Autodesk Inventor part; units mm, degrees
(part 2 of 2)
  arc A205 (-7.2812, 208.5616) -> (-8.6448, 208.5044) centre (-6.6997, 178.392) ccw projected
  arc A206 (-8.6448, 208.5044) -> (-9.6498, 211.2799) centre (-21.0077, 205.5976) ccw projected
  arc A207 (-9.6498, 211.2799) -> (-10.6519, 211.1746) centre (-6.6997, 178.392) ccw projected
  arc A208 (-10.6519, 211.1746) -> (-11.0579, 208.2508) centre (1.6392, 207.9779) ccw projected
  arc A209 (-11.0579, 208.2508) -> (-12.4036, 208.0232) centre (-6.6997, 178.392) ccw projected
  arc A210 (-12.4036, 208.0232) -> (-13.7485, 210.6508) centre (-24.3047, 203.5899) ccw projected
  arc A211 (-13.7485, 210.6508) -> (-14.7295, 210.4207) centre (-6.6997, 178.392) ccw projected
  arc A212 (-14.7295, 210.4207) -> (-14.7658, 207.4691) centre (-2.1347, 208.7898) ccw projected
  arc A213 (-14.7658, 207.4691) -> (-16.0724, 207.0746) centre (-6.6997, 178.392) ccw projected
  arc A214 (-16.0724, 207.0746) -> (-17.736, 209.513) centre (-27.324, 201.1847) ccw projected
  arc A215 (-17.736, 209.513) -> (-18.6805, 209.1618) centre (-6.6997, 178.392) ccw projected
  arc A216 (-18.6805, 209.1618) -> (-18.3466, 206.2289) centre (-5.9806, 209.1222) ccw projected
  arc A217 (-18.3466, 206.2289) -> (-19.5934, 205.6738) centre (-6.6997, 178.392) ccw projected
  arc A218 (-19.5934, 205.6738) -> (-21.5495, 207.8844) centre (-30.018, 198.4201) ccw projected
  arc A219 (-21.5495, 207.8844) -> (-22.4425, 207.4176) centre (-6.6997, 178.392) ccw projected
  arc A220 (-22.4425, 207.4176) -> (-21.7436, 204.5496) centre (-9.8377, 208.9701) ccw projected
  arc A221 (-21.7436, 204.5496) -> (-22.911, 203.8426) centre (-6.6997, 178.392) ccw projected
  arc A222 (-22.911, 203.8426) -> (-25.1288, 205.7907) centre (-32.3443, 195.3396) ccw projected
  arc A223 (-25.1288, 205.7907) -> (-25.9562, 205.2156) centre (-6.6997, 178.392) ccw projected
  arc A224 (-25.9562, 205.2156) -> (-24.9034, 202.4579) centre (-13.6455, 208.3356) ccw projected
  arc A225 (-24.9034, 202.4579) -> (-25.973, 201.6101) centre (-6.6997, 178.392) ccw projected
  arc A226 (-25.973, 201.6101) -> (-28.4175, 203.2649) centre (-34.2662, 191.9918) ccw projected
  arc A227 (-28.4175, 203.2649) -> (-29.1663, 202.5906) centre (-6.6997, 178.392) ccw projected
  arc A228 (-29.1663, 202.5906) -> (-27.7761, 199.9866) centre (-17.3436, 207.229) ccw projected
  arc A229 (-27.7761, 199.9866) -> (-28.731, 199.0115) centre (-6.6997, 178.392) ccw projected
  arc A230 (-28.731, 199.0115) -> (-31.3636, 200.3468) centre (-35.7534, 188.4296) ccw projected
  arc A231 (-31.3636, 200.3468) -> (-32.022, 199.584) centre (-6.6997, 178.392) ccw projected
  arc A232 (-32.022, 199.584) -> (-30.3165, 197.1747) centre (-20.8739, 205.6676) ccw projected
  arc A233 (-30.3165, 197.1747) -> (-31.1416, 196.0876) centre (-6.6997, 178.392) ccw projected
  arc A234 (-31.1416, 196.0876) -> (-33.9208, 197.0825) centre (-36.7823, 184.709) ccw projected
  arc A235 (-33.9208, 197.0825) -> (-34.4784, 196.2432) centre (-6.6997, 178.392) ccw projected
  arc A236 (-34.4784, 196.2432) -> (-32.4844, 194.0667) centre (-24.1807, 203.676) ccw projected
  arc A237 (-32.4844, 194.0667) -> (-33.1668, 192.8847) centre (-6.6997, 178.392) ccw projected
  arc A238 (-33.1668, 192.8847) -> (-36.0487, 193.5234) centre (-37.3369, 180.8889) ccw projected
  arc A239 (-36.0487, 193.5234) -> (-36.4967, 192.6208) centre (-6.6997, 178.392) ccw projected
  arc A240 (-36.4967, 192.6208) -> (-34.2456, 190.7114) centre (-27.2118, 201.2857) ccw projected
  arc A241 (-34.2456, 190.7114) -> (-34.7745, 189.4533) centre (-6.6997, 178.392) ccw projected
  arc A242 (-34.7745, 189.4533) -> (-37.7137, 189.7257) centre (-37.4082, 177.0293) ccw projected
  arc A243 (-37.7137, 189.7257) -> (-38.0451, 188.7741) centre (-6.6997, 178.392) ccw projected
  arc A244 (-38.0451, 188.7741) -> (-35.5724, 187.1618) centre (-29.9194, 198.5343) ccw projected
  arc A245 (-35.5724, 187.1618) -> (-35.9394, 185.8473) centre (-6.6997, 178.392) ccw projected
  arc A246 (-35.9394, 185.8473) -> (-38.8897, 185.7492) centre (-36.9953, 173.1913) ccw projected
  arc A247 (-38.8897, 185.7492) -> (-39.0992, 184.7636) centre (-6.6997, 178.392) ccw projected
  arc A248 (-39.0992, 184.7636) -> (-36.4439, 183.474) centre (-32.2608, 195.4653) ccw projected
  arc A249 (-36.4439, 183.474) -> (-36.6433, 182.1238) centre (-6.6997, 178.392) ccw projected
  arc A250 (-36.6433, 182.1238) -> (-39.558, 181.6567) centre (-36.1046, 169.4353) ccw projected
  arc A251 (-39.558, 181.6567) -> (-39.6423, 180.6526) centre (-6.6997, 178.392) ccw projected
  arc A252 (-39.6423, 180.6526) -> (-36.8463, 179.706) centre (-34.1991, 192.127) ccw projected
  arc A253 (-36.8463, 179.706) -> (-36.8749, 178.3415) centre (-6.6997, 178.392) ccw projected
  arc A254 (-36.8749, 178.3415) -> (-39.708, 177.5128) centre (-34.7502, 165.8205) ccw projected
  arc A255 (-39.708, 177.5128) -> (-39.6658, 176.506) centre (-6.6997, 178.392) ccw projected
  arc A256 (-39.6658, 176.506) -> (-36.7733, 175.9172) centre (-35.7037, 188.5721) ccw projected
  arc A257 (-36.7733, 175.9172) -> (-36.6306, 174.5599) centre (-6.6997, 178.392) ccw projected
  arc A258 (-36.6306, 174.5599) -> (-39.3376, 173.3827) centre (-32.9533, 162.404) ccw projected
  arc A259 (-39.3376, 173.3827) -> (-39.1695, 172.3891) centre (-6.6997, 178.392) ccw projected
  arc A260 (-39.1695, 172.3891) -> (-36.226, 172.1675) centre (-36.7509, 184.8567) ccw projected
  arc A261 (-36.226, 172.1675) -> (-35.9143, 170.8388) centre (-6.6997, 178.392) ccw projected
  arc A262 (-35.9143, 170.8388) -> (-38.4524, 169.3316) centre (-30.7425, 159.2396) ccw projected
  arc A263 (-38.4524, 169.3316) -> (-38.1611, 168.3669) centre (-6.6997, 178.392) ccw projected
  arc A264 (-38.1611, 168.3669) -> (-35.2131, 168.516) centre (-37.3242, 181.0393) ccw projected
  arc A265 (-35.2131, 168.516) -> (-34.7373, 167.2368) centre (-6.6997, 178.392) ccw projected
  arc A266 (-34.7373, 167.2368) -> (-37.0664, 165.4233) centre (-28.1525, 156.3773) ccw projected
  arc A267 (-37.0664, 165.4233) -> (-36.6566, 164.5028) centre (-6.6997, 178.392) ccw projected
  arc A268 (-36.6566, 164.5028) -> (-33.7504, 165.0202) centre (-37.4145, 177.1802) ccw projected
  arc A269 (-33.7504, 165.0202) -> (-33.1181, 163.8107) centre (-6.6997, 178.392) ccw projected
  arc A270 (-33.1181, 163.8107) -> (-35.2016, 161.7197) centre (-25.2242, 153.8621) ccw projected
  arc A271 (-35.2016, 161.7197) -> (-34.6796, 160.8577) centre (-6.6997, 178.392) ccw projected
  arc A272 (-34.6796, 160.8577) -> (-31.8612, 161.7353) centre (-37.0205, 173.3401) ccw projected
  arc A273 (-31.8612, 161.7353) -> (-31.0823, 160.6146) centre (-6.6997, 178.392) ccw projected
  arc A274 (-31.0823, 160.6146) -> (-32.8872, 158.2789) centre (-22.0037, 151.7338) ccw projected
  arc A275 (-32.8872, 158.2789) -> (-32.2613, 157.4892) centre (-6.6997, 178.392) ccw projected
  arc A276 (-32.2613, 157.4892) -> (-29.5752, 158.7131) centre (-36.1482, 169.5798) ccw projected
  arc A277 (-29.5752, 158.7131) -> (-28.6619, 157.6989) centre (-6.6997, 178.392) ccw projected
  arc A278 (-28.6619, 157.6989) -> (-30.1599, 155.1553) centre (-18.5419, 150.0259) ccw projected
  arc A279 (-30.1599, 155.1553) -> (-29.44, 154.4503) centre (-6.6997, 178.392) ccw projected
  arc A280 (-29.44, 154.4503) -> (-26.9284, 156.0012) centre (-34.8116, 165.9584) ccw projected
  arc A281 (-26.9284, 156.0012) -> (-25.8952, 155.1094) centre (-6.6997, 178.392) ccw projected
  arc A282 (-25.8952, 155.1094) -> (-27.0626, 152.3982) centre (-14.8933, 148.7654) ccw projected
  arc A283 (-27.0626, 152.3982) -> (-26.26, 151.789) centre (-6.6997, 178.392) ccw projected
  arc A284 (-26.26, 151.789) -> (-23.9626, 153.6424) centre (-33.0315, 162.5331) ccw projected
  arc A285 (-23.9626, 153.6424) -> (-22.8258, 152.8872) centre (-6.6997, 178.392) ccw projected
  arc A286 (-22.8258, 152.8872) -> (-23.6442, 150.051) centre (-11.1155, 147.9721) ccw projected
  arc A287 (-23.6442, 150.051) -> (-22.7715, 149.5472) centre (-6.6997, 178.392) ccw projected
  arc A288 (-22.7715, 149.5472) -> (-20.7245, 151.674) centre (-30.8363, 159.3579) ccw projected
  arc A289 (-20.7245, 151.674) -> (-19.502, 151.0672) centre (-6.6997, 178.392) ccw projected
  arc A290 (-19.502, 151.0672) -> (-19.9585, 148.1508) centre (-7.268, 147.6585) ccw projected
  arc A291 (-19.9585, 148.1508) -> (-19.0296, 147.7603) centre (-6.6997, 178.392) ccw projected
  arc A292 (-19.0296, 147.7603) -> (-17.2653, 150.1269) centre (-28.2603, 156.4829) ccw projected
  arc A293 (-17.2653, 150.1269) -> (-15.9764, 149.6781) centre (-6.6997, 178.392) ccw projected
  arc A294 (-15.9764, 149.6781) -> (-16.0637, 146.7275) centre (-3.4116, 147.8296) ccw projected
  arc A295 (-16.0637, 146.7275) -> (-15.0932, 146.4565) centre (-6.6997, 178.392) ccw projected
  arc A296 (-15.0932, 146.4565) -> (-13.6394, 149.0256) centre (-25.3444, 153.9534) ccw projected
  arc A297 (-13.6394, 149.0256) -> (-12.3044, 148.7418) centre (-6.6997, 178.392) ccw projected
  arc A298 (-12.3044, 148.7418) -> (-12.0213, 145.8036) centre (0.3929, 148.4827) ccw projected
  arc A299 (-12.0213, 145.8036) -> (-11.0244, 145.6564) centre (-6.6997, 178.392) ccw projected
  arc A300 (-11.0244, 145.6564) -> (-9.9041, 148.3874) centre (-22.1344, 151.8093) ccw projected
  arc A301 (-9.9041, 148.3874) -> (-8.5441, 148.2732) centre (-6.6997, 178.392) ccw projected
  arc A302 (-8.5441, 148.2732) -> (-7.8949, 145.3936) centre (4.0856, 149.6075) ccw projected
  arc A303 (-7.8949, 145.3936) -> (-6.8875, 145.3725) centre (-6.6997, 178.392) ccw projected
  arc A304 (-6.8875, 145.3725) -> (-6.1183, 148.2224) centre (-18.681, 150.0844) ccw projected
  arc A305 (-6.1183, 148.2224) -> (-4.7547, 148.2795) centre (-6.6997, 178.392) ccw projected
  arc A306 (-4.7547, 148.2795) -> (-3.7497, 145.504) centre (7.6082, 151.1863) ccw projected
  arc A307 (-3.7497, 145.504) -> (-2.7476, 145.6093) centre (-6.6997, 178.392) ccw projected
  arc A308 (-2.7476, 145.6093) -> (-2.3416, 148.5331) centre (-15.0387, 148.806) ccw projected
  arc A309 (-2.3416, 148.5331) -> (-0.9959, 148.7607) centre (-6.6997, 178.392) ccw projected
  arc A310 (-0.9959, 148.7607) -> (0.349, 146.1331) centre (10.9052, 153.1941) ccw projected
  arc A311 (0.349, 146.1331) -> (1.33, 146.3632) centre (-6.6997, 178.392) ccw projected
  arc A312 (1.33, 146.3632) -> (1.3663, 149.3148) centre (-11.2648, 147.9941) ccw projected
  arc A313 (1.3663, 149.3148) -> (2.6729, 149.7093) centre (-6.6997, 178.392) ccw projected
  arc A314 (2.6729, 149.7093) -> (4.3365, 147.2709) centre (13.9245, 155.5992) ccw projected
  arc A315 (4.3365, 147.2709) -> (5.281, 147.6221) centre (-6.6997, 178.392) ccw projected
  arc A316 (5.281, 147.6221) -> (4.9471, 150.555) centre (-7.4189, 147.6617) ccw projected
  arc A317 (4.9471, 150.555) -> (6.1939, 151.1101) centre (-6.6997, 178.392) ccw projected
  arc A318 (6.1939, 151.1101) -> (8.15, 148.8995) centre (16.6185, 158.3639) ccw projected
  arc A319 (8.15, 148.8995) -> (9.043, 149.3663) centre (-6.6997, 178.392) ccw projected
  arc A320 (9.043, 149.3663) -> (8.3441, 152.2343) centre (-3.5618, 147.8139) ccw projected
  arc A321 (8.3441, 152.2343) -> (9.5115, 152.9413) centre (-6.6997, 178.392) ccw projected
  arc A322 (9.5115, 152.9413) -> (11.7293, 150.9932) centre (18.9448, 161.4443) ccw projected
  arc A323 (11.7293, 150.9932) -> (12.5567, 151.5683) centre (-6.6997, 178.392) ccw projected
  arc A324 (12.5567, 151.5683) -> (11.5039, 154.326) centre (0.246, 148.4483) ccw projected
  arc A325 (11.5039, 154.326) -> (12.5735, 155.1738) centre (-6.6997, 178.392) ccw projected
  arc A326 (12.5735, 155.1738) -> (15.018, 153.519) centre (20.8667, 164.7921) ccw projected
  arc A327 (15.018, 153.519) -> (15.7668, 154.1933) centre (-6.6997, 178.392) ccw projected
  arc A328 (15.7668, 154.1933) -> (14.3766, 156.7973) centre (3.9441, 149.5549) ccw projected
  arc A329 (14.3766, 156.7973) -> (15.3315, 157.7724) centre (-6.6997, 178.392) ccw projected
  arc A330 (15.3315, 157.7724) -> (17.9641, 156.4371) centre (22.3539, 168.3543) ccw projected
  arc A331 (17.9641, 156.4371) -> (18.6225, 157.1999) centre (-6.6997, 178.392) ccw projected
  arc A332 (18.6225, 157.1999) -> (16.917, 159.6092) centre (7.4744, 151.1163) ccw projected
  arc A333 (16.917, 159.6092) -> (17.7421, 160.6963) centre (-6.6997, 178.392) ccw projected
  arc A334 (17.7421, 160.6963) -> (20.5213, 159.7014) centre (23.3828, 172.0749) ccw projected
  arc A335 (20.5213, 159.7014) -> (21.0789, 160.5407) centre (-6.6997, 178.392) ccw projected
  arc A336 (21.0789, 160.5407) -> (19.0849, 162.7172) centre (10.7812, 153.1079) ccw projected
  arc A337 (19.0849, 162.7172) -> (19.7673, 163.8992) centre (-6.6997, 178.392) ccw projected
  arc A338 (19.7673, 163.8992) -> (22.6492, 163.2605) centre (23.9374, 175.895) ccw projected
  arc A339 (22.6492, 163.2605) -> (23.0972, 164.1631) centre (-6.6997, 178.392) ccw projected
  arc A340 (23.0972, 164.1631) -> (20.8461, 166.0725) centre (13.8123, 155.4982) ccw projected
  arc A341 (20.8461, 166.0725) -> (21.375, 167.3307) centre (-6.6997, 178.392) ccw projected
  line L3 (61.9125, 171.704) -> (29.446, 168.6111) projected
  circle A342 centre (-6.6997, 178.392) radius 37.4457
  circle A343 centre (36.5125, 146.05) radius 28.194
  point P0 (0, 0)
  point P1 (50.3685, 170.6043)
  point P2 (30.4357, 173.5813)
  dimension "d10" = 56.388
  constraints: 2 coincident, 1 centre point, 3 other
  measures "d10" diameter of A343
extrude "Extrusion2" cut sketch "Sketch2" against normal blind 12.7 contours A343 L3 A342
sketch "Sketch3" plane through (0, 0, 0) normal (0, 0, -1) x (-1, 0, 0)
  arc A0 (50.3685, 170.6043) -> (30.4357, 173.5813) centre (36.5125, 146.05) ccw projected
  line L0 (61.9125, 171.704) -> (50.3685, 170.6043) projected
  line L1 (61.9125, 190.5) -> (61.9125, 171.704) projected
  arc A1 (40.9534, 289.0612) -> (-0.498, 261.4395) centre (17.4625, 279.4) ccw projected
  circle A2 centre (17.4625, 279.4) radius 15.9004 projected
  circle A3 centre (40.0964, 179.0237) radius 3.175 projected
  circle A4 centre (52.7964, 180.2336) radius 3.175 projected
  circle A5 centre (40.0964, 182.1987) radius 3.175
  arc A6 (29.446, 168.6111) -> (30.4357, 173.5813) centre (-6.6997, 178.392) ccw projected
  point P0 (0, 0)
  point P1 (42.8461, 180.6112)
  point P2 (37.3468, 180.6112)
  dimension "d13" = 6.35
  constraints: 1 centre point, 4 other
  measures "d13" diameter of A5
extrude "Extrusion3" add sketch "Sketch3" against normal blind 12.7 contours A3 A5 picked at (39.9369, 176.9303)
extrude "Extrusion4" cut sketch "Sketch3" against normal blind 12.7 contours A3 A5 picked at (39.9369, 184.2921)
fillet "Fillet1" radius 6.35 2 edges at (-50.3685, 170.6043, 6.35) (-61.9125, 171.704, 6.35)
sketch "Sketch4" plane through (0, 0, 0) normal (0, 0, -1) x (-1, 0, 0)
  arc A0 (56.1647, 171.1564) -> (61.9125, 177.4778) centre (55.5625, 177.4778) ccw projected
  line L0 (61.9125, 190.5) -> (61.9125, 177.4778) projected
  spline S0 degree 2 poles (40.9534, 289.0612) (61.9125, 238.0996) (61.9125, 190.5) knots 0 0 0 1 1 1
  arc A1 (40.9534, 289.0612) -> (-0.498, 261.4395) centre (17.4625, 279.4) ccw projected
  spline S1 degree 3 poles (29.446, 168.6111) (27.6192, 182.9318) (26.9203, 234.0212) (-0.498, 261.4395) knots 0 0 0 0 1 1 1 1
  arc A2 (48.8612, 171.3959) -> (30.4357, 173.5813) centre (36.5125, 146.05) ccw projected
  arc A3 (48.8612, 171.3959) -> (52.2446, 170.783) centre (51.6424, 177.1044) ccw projected
  line L1 (56.1647, 171.1564) -> (52.2446, 170.783) projected
  circle A4 centre (17.4625, 279.4) radius 15.9004 projected
  circle A5 centre (40.0964, 182.1987) radius 3.175 projected
  circle A6 centre (52.7964, 180.2336) radius 3.175 projected
  line L2 (55.5625, 190.5) -> (55.5625, 177.4778)
  line L3 (55.5625, 177.4778) -> (51.6424, 177.1044)
  arc A7 (51.6424, 177.1044) -> (34.6938, 180.5461) centre (36.5125, 146.05) ccw
  arc A8 (35.0807, 286.6459) -> (3.9921, 265.9296) centre (17.4625, 279.4) ccw
  circle A9 centre (17.4625, 279.4) radius 40.9661
  circle A10 centre (40.0964, 182.1987) radius 9.525
  circle A11 centre (52.7964, 180.2336) radius 9.525
  line L4 (33.448, 192.2945) -> (55.5625, 190.5)
  line L5 (47.1822, 251.2049) -> (33.448, 192.2945)
  line L6 (50.6373, 249.2445) -> (38.1622, 195.7345)
  line L7 (38.1622, 195.7345) -> (59.3725, 194.0133)
  line L8 (59.3725, 194.0133) -> (59.3725, 174.0135)
  line L9 (59.3725, 174.0135) -> (50.9032, 173.2067)
  arc A12 (50.9032, 173.2067) -> (37.3679, 176.7721) centre (36.5125, 146.05) ccw
  line L10 (44.4515, 250.6867) -> (30.3031, 189.9997)
  line L11 (30.3031, 189.9997) -> (53.0208, 188.1562)
  line L12 (53.0208, 188.1562) -> (53.0208, 179.7889)
  line L13 (53.0208, 179.7889) -> (52.0994, 179.7012)
  arc A13 (52.0994, 179.7012) -> (37.5447, 183.1214) centre (36.5125, 146.05) ccw
  arc A14 (29.446, 168.6111) -> (30.4357, 173.5813) centre (-6.6997, 178.392) ccw projected
  spline S2 degree 5 poles (34.6938, 180.5461) (34.5354, 182.2782) (34.3709, 184.0098) (34.1972, 185.7405) (33.7041, 190.3635) (33.1253, 194.9769) (32.7234, 197.8591) (31.7796, 203.9538) (30.6206, 210.0115) (29.9427, 213.1978) (28.398, 219.7282) (26.5193, 226.1708) (25.4561, 229.457) (23.0874, 236.0456) (20.2467, 242.4451) (18.6762, 245.628) (15.2193, 251.9029) (11.1499, 257.7995) (8.9323, 260.6586) (6.5449, 263.3768) (3.9921, 265.9296) knots 0 0 0 0 0 0 0.093954 0.093954 0.093954 0.25113 0.25113 0.25113 0.427044 0.427044 0.427044 0.6135 0.6135 0.6135 0.804991 0.804991 0.804991 1 1 1 1 1 1
  spline S3 degree 5 poles (35.0807, 286.6459) (42.6076, 268.3457) (48.7539, 249.483) (53.2276, 230.0774) (55.5632, 210.2861) (55.5625, 190.5) knots 0 0 0 0 0 0 1 1 1 1 1 1
  point P0 (0, 0)
  point P1 (32.4777, 199.3272)
  point P2 (43.8377, 248.054)
  point P3 (21.8585, 238.6704)
  point P4 (55.5277, 194.3253)
  point P5 (49.2184, 243.1584)
  dimension "d19" = 6.35
  dimension "d20" = 19.05
  dimension "d21" = 19.05
  dimension "d22" = 3.81
  constraints: 24 end point, 8 point on circle, 6 centre point, 3 coincident, 3 concentric, 1 tangent, 23 other
  measures "d20" diameter of A10
  measures "d21" diameter of A11
  measures "d22" distance between parallel lines of L5 L6
extrude "Extrusion5" cut sketch "Sketch4" against normal blind 12.7 contours L7 L6 S3 | L10 S2 A9
fillet "Fillet2" radius 3.175 6 edges at (-43.8377, 248.054, 6.35) (-49.2184, 243.1584, 6.35) (-21.8585, 238.6704, 6.35) (-32.4777, 199.3272, 6.35) (-38.1622, 195.7345, 6.35) (-55.5278, 194.3253, 6.35)
thread "Thread1" size "1/4-20 UNC" class "2B" standard "ANSI Unified Screw Threads" full length
thread "Thread2" size "8-32 UNC" class "2B" standard "ANSI Unified Screw Threads" full length
sketch "Sketch5" plane through (0, 0, 0) normal (0, 0, -1) x (-1, 0, 0)
  circle A0 centre (52.7964, 180.2336) radius 3.175 projected
  circle A1 centre (52.7964, 180.2336) radius 2.413
  circle A2 centre (40.0964, 182.1987) radius 3.175 projected
  circle A3 centre (40.0964, 182.1987) radius 2.413
  point P0 (0, 0)
  dimension "d30" = 4.826
  dimension "d31" = 4.826
  constraints: 2 centre point, 2 coincident
  measures "d30" diameter of A1
  measures "d31" diameter of A3
extrude "Extrusion6" add sketch "Sketch5" against normal blind 12.7
thread "Thread3" size "10-24 UNC" class "2B" standard "ANSI Unified Screw Threads" full length
thread "Thread4" size "10-24 UNC" class "2B" standard "ANSI Unified Screw Threads" full length
sketch "Sketch6" plane through (0, 0, 12.7) normal (0, 0, 1) x (1, 0, 0)
  circle A0 centre (-40.0964, 182.1987) radius 2.413 projected
  circle A1 centre (-52.7964, 180.2336) radius 2.413 projected
  line L0 (-35.8997, 214.0052) -> (-41.9802, 240.0866) projected
  arc A2 (-37.347, 243.5834) -> (-41.9802, 240.0866) centre (-38.8881, 240.8075) ccw projected
  arc A3 (-37.347, 243.5834) -> (-25.6845, 239.2675) centre (-17.4625, 279.4) ccw projected
  line L1 (-45.9336, 229.0686) -> (-38.9986, 199.3221) projected
  arc A4 (-41.8339, 195.4366) -> (-38.9986, 199.3221) centre (-42.0907, 198.6012) ccw projected
  line L2 (-41.8339, 195.4366) -> (-52.0034, 194.6113) projected
  arc A5 (-61.9125, 177.4778) -> (-56.1647, 171.1564) centre (-55.5625, 177.4778) ccw projected
  line L3 (-56.1647, 171.1564) -> (-52.2446, 170.783) projected
  arc A6 (-52.2446, 170.783) -> (-48.8612, 171.3959) centre (-51.6424, 177.1044) ccw projected
  arc A7 (-30.4357, 173.5813) -> (-48.8612, 171.3959) centre (-36.5125, 146.05) ccw projected
  arc A8 (0.498, 261.4395) -> (-40.9534, 289.0612) centre (-17.4625, 279.4) ccw projected
  line L4 (-61.9125, 190.5) -> (-61.9125, 177.4778) projected
  circle A9 centre (-17.4625, 279.4) radius 15.9004 projected
  circle A10 centre (-52.7964, 180.2336) radius 1.27
  circle A11 centre (-40.0964, 182.1987) radius 1.27
  arc A12 (-30.4357, 173.5813) -> (-29.446, 168.6111) centre (6.6997, 178.392) ccw projected
  point P0 (0, 0)
  dimension "d38" = 2.54
  dimension "d39" = 2.54
  constraints: 2 centre point, 2 coincident, 8 other
  measures "d38" diameter of A10
  measures "d39" diameter of A11
extrude "Extrusion7" add sketch "Sketch6" against normal up to surface (12.7 mm away) contours A0 | A1
sketch "Sketch7" plane through (0, 0, 12.7) normal (0, 0, 1) x (1, 0, 0)
  circle A0 centre (-40.0964, 182.1987) radius 1.27 projected
  circle A1 centre (-52.7964, 180.2336) radius 1.27 projected
  line L0 (-35.8997, 214.0052) -> (-41.9802, 240.0866) projected
  arc A2 (-37.347, 243.5834) -> (-41.9802, 240.0866) centre (-38.8881, 240.8075) ccw projected
  arc A3 (-37.347, 243.5834) -> (-25.6845, 239.2675) centre (-17.4625, 279.4) ccw projected
  line L1 (-45.9336, 229.0686) -> (-38.9986, 199.3221) projected
  arc A4 (-41.8339, 195.4366) -> (-38.9986, 199.3221) centre (-42.0907, 198.6012) ccw projected
  line L2 (-41.8339, 195.4366) -> (-52.0034, 194.6113) projected
  arc A5 (-61.9125, 177.4778) -> (-56.1647, 171.1564) centre (-55.5625, 177.4778) ccw projected
  line L3 (-56.1647, 171.1564) -> (-52.2446, 170.783) projected
  arc A6 (-52.2446, 170.783) -> (-48.8612, 171.3959) centre (-51.6424, 177.1044) ccw projected
  arc A7 (-30.4357, 173.5813) -> (-48.8612, 171.3959) centre (-36.5125, 146.05) ccw projected
  arc A8 (0.498, 261.4395) -> (-40.9534, 289.0612) centre (-17.4625, 279.4) ccw projected
  line L4 (-61.9125, 190.5) -> (-61.9125, 177.4778) projected
  circle A9 centre (-17.4625, 279.4) radius 15.9004 projected
  circle A10 centre (-17.4625, 279.4) radius 15.24
  arc A11 (-30.4357, 173.5813) -> (-29.446, 168.6111) centre (6.6997, 178.392) ccw projected
  point P0 (0, 0)
  dimension "d42" = 30.48
  constraints: 1 centre point, 1 coincident, 8 other
  measures "d42" diameter of A10
extrude "Extrusion8" add sketch "Sketch7" against normal blind 12.7 contours A9
body "Solid1"
